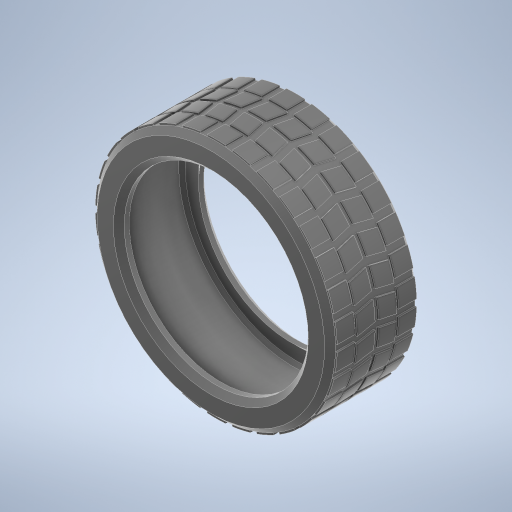
# Autodesk Inventor part: Karet Roda Mainan
Saved by Autodesk Inventor 2023 (Build 270158000, 158)
## iProperties
Created: 2023-08-24
Part Number: Karet Roda Mainan
Material: Rubber
Document SubType Name: Modeling
Designer: LENOVO IP320-14IKB
Density: 0.93 g/cm^3
Appearance: Smooth - Black
Author: LENOVO IP320-14IKB
Autodesk Inventor part; units mm, degrees
ref_plane "YZ Plane" through (0, 0, 0) normal (1, 0, 0) x (0, 1, 0)
ref_plane "XY Plane" through (0, 0, 0) normal (0, 0, 1) x (1, 0, 0)
sketch "Sketch1" plane through (0, 0, 0) normal (0, 0, 1) x (1, 0, 0)
  circle A0 centre (0, 0) radius 33
  circle A1 centre (0, 0) radius 25.5
  dimension "d0" = 66
  dimension "d1" = 51
  constraints: 2 centre point, 2 coincident
  measures "d0" diameter of A0
  measures "d1" diameter of A1
extrude "Extrusion1" add sketch "Sketch1" along normal blind 25
chamfer "Chamfer1" distance 1.5 angle 45 4 edges at (-25.5, 0, 25) (-33, 0, 25) (-33, 0, 0) (-25.5, 0, 0)
shell "Shell1" thickness 1 removed faces 1 at (25.4173, -2.0519, 16.1667)
ref_plane "Work Plane1" through (0, 35, 0) normal (0, 1, 0) x (-1, 0, 0)
sketch "Sketch2" plane through (0, 35, 0) normal (0, 1, 0) x (-1, 0, 0)
  line L0 (2.5, 1.5) -> (-2.5, 1.5)
  line L1 (-2.5, 1.5) -> (-2.5, 6.5)
  line L2 (-2.5, 6.5) -> (2.5, 6.5)
  line L3 (2.5, 6.5) -> (2.5, 1.5)
  line L4 (31.5, 0) -> (-31.5, 0) projected
  line L5 (1.7, 7) -> (-3.3, 7)
  line L6 (-2.3, 12) -> (2.7, 12)
  line L7 (-3.3, 7) -> (-2.3, 12)
  line L8 (2.7, 12) -> (1.7, 7)
  line L9 (5.1784, 12.5) -> (-5.1784, 12.5) construction
  line L10 (2.5, 23.5) -> (-2.5, 23.5)
  line L11 (-2.5, 23.5) -> (-2.5, 18.5)
  line L12 (-2.5, 18.5) -> (2.5, 18.5)
  line L13 (2.5, 18.5) -> (2.5, 23.5)
  line L14 (1.7, 18) -> (-3.3, 18)
  line L15 (-2.3, 13) -> (2.7, 13)
  line L16 (-3.3, 18) -> (-2.3, 13)
  line L17 (2.7, 13) -> (1.7, 18)
  point P0 (0, 0)
  point P1 (0, 1.5)
  point P2 (0, 0)
  point P3 (0, 7)
  point P4 (0, 6.5)
  point P5 (0, 12.5)
  point P6 (0, 23.5)
  point P7 (0, 18)
  point P8 (0, 18.5)
  dimension "d9" = 5
  dimension "d10" = 5
  dimension "d11" = 1.5
  dimension "d14" = 0.5
  dimension "d17" = 5
  dimension "d18" = 12.5
  constraints: 34 end point, 11 symmetric about line, 4 midpoint, 4 parallel, 3 horizontal, 3 vertical alignment, 2 point on line, 1 perpendicular, 2 other
  measures "d9" distance of L1.end L2.end
  measures "d10" distance of L0.end L1.end
  measures "d11" distance between parallel lines of L0 L4
  measures "d14" distance from line of L5 point (0, 6.5)
  measures "d17" distance between parallel lines of L5 L6
  measures "d18" distance between parallel lines of L4 L9
emboss "Emboss1" sketch "Sketch2" operation add depth 0.5 direction (0, 1, 0) wrap yes faces at (32.893, -2.6554, 16.1667)
pattern_circular "Circular Pattern1" count 30 over 360 about axis through (0, 0, 0) along (0, 0, 1) of "Emboss1"
body "Solid1"
